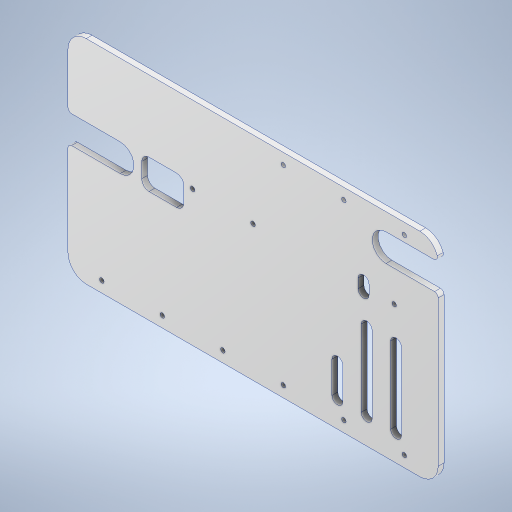
# Autodesk Inventor part: Class-D RevA Board Heatsink
Saved by Autodesk Inventor 2024 (Build 280153000, 153)
## iProperties
Created: 2023-08-05
Part Number: Class-D RevA Board Heatsink
Material: Aluminum 6061
Document SubType Name: Modeling
Designer: Ishaan
Density: 2.7 g/cm^3
Appearance: Aluminum - Flat
Author: Ishaan
Autodesk Inventor part; units mm, degrees
ref_plane "YZ Plane" through (0, 0, 0) normal (1, 0, 0) x (0, 1, 0)
ref_plane "XZ Plane" through (0, 0, 0) normal (0, 1, 0) x (-1, 0, 0)
ref_plane "XY Plane" through (0, 0, 0) normal (0, 0, 1) x (1, 0, 0)
sketch "Sketch1" plane through (0, 0, 0) normal (0, 0, 1) x (1, 0, 0)
  line L0 (-99, -56) -> (99, -56)
  line L1 (99, -56) -> (99, 56)
  line L2 (99, 56) -> (-99, 56)
  line L3 (-99, 56) -> (-99, -56)
  line L4 (-99, -56) -> (99, 56) construction
  line L5 (99, -56) -> (-99, 56) construction
  line L6 (-99, -56) -> (8.25, -56)
  line L7 (8.25, -56) -> (8.25, 20)
  line L8 (8.25, 20) -> (-99, 20)
  line L9 (-99, 20) -> (-99, -56)
  line L10 (8.25, 20) -> (8.25, 56)
  point P0 (0, 0)
  dimension "d0" = 112
  dimension "d1" = 198
  dimension "d3" = 76
  dimension "d50" = 8.25
  constraints: 22 end point, 4 parallel, 3 perpendicular, 2 horizontal, 2 midpoint, 1 point on line
  measures "d0" distance of L0.end L1.end
  measures "d1" distance of L1.end L2.end
  measures "d3" distance of L6.end L7.end
  measures "d50" distance from line of L10 point (0, 0)
extrude "Extrusion1" add sketch "Sketch1" along normal blind 3.175
sketch "Sketch2" plane through (0, 0, 3.175) normal (0, 0, 1) x (1, 0, 0)
  line L0 (-99, -56) -> (99, -56) projected
  line L1 (-99, 56) -> (-99, -56) projected
  line L2 (99, 56) -> (-99, 56) projected
  line L3 (99, -56) -> (99, 56) projected
  line L4 (-16.5, -52) -> (16.5, -52) construction
  line L5 (-49.5, -52) -> (-16.5, -52) construction
  line L6 (8.25, 20) -> (-99, 20) projected
  point P0 (0, 0)
  point P1 (-82.5, -52)
  point P2 (49.5, -52)
  point P3 (-82.5, 52)
  point P4 (-49.5, 52)
  point P5 (-16.5, 52)
  point P6 (16.5, 52)
  point P7 (49.5, 52)
  point P8 (82.5, -52)
  point P9 (82.5, 52)
  point P10 (-33, 16)
  point P11 (0, 16)
  point P12 (0, -52)
  point P13 (-33, -52)
  dimension "d6" = 4
  dimension "d9" = 33
  dimension "d12" = 104
  dimension "d15" = 4
  dimension "d17" = 16.5
  dimension "d18" = 16.5
  dimension "d51" = 4
  constraints: 4 end point, 3 horizontal, 2 midpoint, 2 vertical alignment, 1 coincident, 1 horizontal alignment, 1 vertical, 11 other
  measures "d6" distance from line of point (-82.5, -52) L0
  measures "d9" distance of point (-82.5, -52) L5.start
  measures "d12" distance of point (-82.5, -52) point (-82.5, 52)
  measures "d15" distance from line of L2 point (-82.5, 52)
  measures "d17" distance from line of point (-82.5, -52) L1
  measures "d18" distance from line of point (82.5, -52) L3
  measures "d51" distance from line of L6 point (-33, 16)
hole "Hole1" at (-82.5, -52, 3.175) at (-49.5, -52, 3.175) at (-16.5, -52, 3.175) at (16.5, -52, 3.175) at (49.5, -52, 3.175) at (16.5, 52, 3.175) at (49.5, 52, 3.175) at (82.5, -52, 3.175) at (82.5, 52, 3.175) at (-33, 16, 3.175) at (0, 16, 3.175) direction (0, 0, -1) diameter 2.459 end through all thread size "M3x0.5" class "6H" standard "ANSI Metric M Profile"
fillet "Fillet4" radius 8 4 edges at (99, -56, 1.5875) (-99, -56, 1.5875) (-99, 56, 1.5875) (99, 56, 1.5875)
sketch "Sketch6" plane through (0, 0, 3.175) normal (0, 0, 1) x (1, 0, 0)
  arc A0 (99, 48) -> (91, 56) centre (91, 48) ccw projected
  line L0 (91, 56) -> (-91, 56) projected
  arc A1 (-91, 56) -> (-99, 48) centre (-91, 48) ccw projected
  line L1 (-99, 48) -> (-99, -48) projected
  arc A2 (-99, -48) -> (-91, -56) centre (-91, -48) ccw projected
  line L2 (-91, -56) -> (91, -56) projected
  arc A3 (91, -56) -> (99, -48) centre (91, -48) ccw projected
  line L3 (99, -48) -> (99, 48) projected
  circle A4 centre (0, 16) radius 1.2295 projected
  circle A5 centre (-33, 16) radius 1.2295 projected
  circle A6 centre (82.5, 52) radius 1.2295 projected
  circle A7 centre (82.5, -52) radius 1.2295 projected
  circle A8 centre (49.5, 52) radius 1.2295 projected
  circle A9 centre (16.5, 52) radius 1.2295 projected
  circle A10 centre (49.5, -52) radius 1.2295 projected
  circle A11 centre (16.5, -52) radius 1.2295 projected
  circle A12 centre (-16.5, -52) radius 1.2295 projected
  circle A13 centre (-49.5, -52) radius 1.2295 projected
  circle A14 centre (-82.5, -52) radius 1.2295 projected
  line L4 (-91, 58) -> (91, 58)
  arc A15 (101, 48) -> (91, 58) centre (91, 48) ccw
  line L5 (101, 48) -> (101, -48)
  arc A16 (91, -58) -> (101, -48) centre (91, -48) ccw
  line L6 (91, -58) -> (-91, -58)
  arc A17 (-101, -48) -> (-91, -58) centre (-91, -48) ccw
  line L7 (-101, -48) -> (-101, 48)
  arc A18 (-91, 58) -> (-101, 48) centre (-91, 48) ccw
  point P0 (0, 0)
  dimension "d53" = 2
  constraints: 8 end point, 8 point on circle, 4 centre point, 7 other
  measures "d53" distance between parallel lines of L0 L4
extrude "Extrusion3" add sketch "Sketch6" against normal up to surface (3.175 mm away) contours L4 A15 L5 A16 L6 A17 L7 A18
sketch "Sketch7" plane through (0, 0, 0) normal (0, 0, -1) x (-1, 0, 0)
  circle A0 centre (-91.5, 41) radius 2.0701 projected
  circle A1 centre (-72.5, 41) radius 2.0701 projected
  circle A2 centre (72.5, 11) radius 2.0701 projected
  circle A3 centre (91.5, 11) radius 2.0701 projected
  line L0 (-72.5, 41) -> (-91.5, 41) construction
  line L1 (-72.5, 48.5) -> (-91.5, 48.5)
  line L2 (-91.5, 33.5) -> (-72.5, 33.5)
  arc A4 (-72.5, 33.5) -> (-72.5, 48.5) centre (-72.5, 41) ccw
  arc A5 (-91.5, 48.5) -> (-91.5, 33.5) centre (-91.5, 41) ccw
  line L3 (-91.5, 48.5) -> (-101, 48.5)
  line L4 (-101, 48.5) -> (-101, 33.5)
  line L5 (-101, 33.5) -> (-91.5, 33.5)
  line L6 (-91.5, 33.5) -> (-91.5, 48.5)
  line L7 (-101, 48) -> (-101, -48) projected
  line L8 (72.5, 11) -> (91.5, 11) construction
  line L9 (72.5, 3.5) -> (91.5, 3.5)
  line L10 (91.5, 18.5) -> (72.5, 18.5)
  arc A6 (72.5, 18.5) -> (72.5, 3.5) centre (72.5, 11) ccw
  arc A7 (91.5, 3.5) -> (91.5, 18.5) centre (91.5, 11) ccw
  line L11 (91.5, 18.5) -> (101, 18.5)
  line L12 (101, 18.5) -> (101, 3.5)
  line L13 (101, 3.5) -> (91.5, 3.5)
  line L14 (91.5, 3.5) -> (91.5, 18.5)
  line L15 (101, -48) -> (101, 48) projected
  point P0 (0, 0)
  point P1 (-82, 41)
  point P2 (82, 11)
  dimension "d56" = 15
  constraints: 32 end point, 8 point on circle, 8 tangent, 6 parallel, 4 centre point, 4 horizontal, 2 midpoint, 2 perpendicular, 1 collinear, 1 equal radius, 1 point on line
  measures "d56" diameter of A5
extrude "Extrusion4" cut sketch "Sketch7" against normal through all contours A0 L6 | A0 L6 L1 A4 L2 | L6 A0 | A0 L6 A5 | A5 L5 L4 L3 | A1 | A2 | A3 L14 | A3 L14 A7 | L14 A3 | A3 L14 L9 A6 L10 | L11 L12 L13 A7
sketch "Sketch8" plane through (0, 0, 0) normal (0, 0, -1) x (-1, 0, 0)
  circle A0 centre (56.75, 6.9) radius 0.75 projected
  circle A1 centre (41.75, 15.1) radius 0.75 projected
  circle A2 centre (-46, -43.54) radius 0.5 projected
  circle A3 centre (-46, -26.46) radius 0.5 projected
  circle A4 centre (-62, -43.54) radius 0.5 projected
  circle A5 centre (-62, -1.875) radius 0.5 projected
  circle A6 centre (-78, -43.54) radius 0.5 projected
  circle A7 centre (-78, -1.875) radius 0.5 projected
  line L0 (-78, -43.54) -> (-78, -1.875) construction
  line L1 (-75, -43.54) -> (-75, -1.875)
  line L2 (-81, -1.875) -> (-81, -43.54)
  arc A8 (-81, -43.54) -> (-75, -43.54) centre (-78, -43.54) ccw
  arc A9 (-75, -1.875) -> (-81, -1.875) centre (-78, -1.875) ccw
  line L3 (-62, -43.54) -> (-62, -1.875) construction
  line L4 (-59, -43.54) -> (-59, -1.875)
  line L5 (-65, -1.875) -> (-65, -43.54)
  arc A10 (-65, -43.54) -> (-59, -43.54) centre (-62, -43.54) ccw
  arc A11 (-59, -1.875) -> (-65, -1.875) centre (-62, -1.875) ccw
  line L6 (-46, -43.54) -> (-46, -26.46) construction
  line L7 (-49, -43.54) -> (-49, -26.46)
  line L8 (-43, -26.46) -> (-43, -43.54)
  arc A12 (-49, -43.54) -> (-43, -43.54) centre (-46, -43.54) ccw
  arc A13 (-43, -26.46) -> (-49, -26.46) centre (-46, -26.46) ccw
  line L9 (41.75, 19.1) -> (56.75, 19.1)
  line L10 (60.75, 15.1) -> (60.75, 6.9)
  line L11 (56.75, 2.9) -> (41.75, 2.9)
  line L12 (37.75, 6.9) -> (37.75, 15.1)
  arc A14 (41.75, 19.1) -> (37.75, 15.1) centre (41.75, 15.1) ccw
  arc A15 (56.75, 2.9) -> (60.75, 6.9) centre (56.75, 6.9) ccw
  arc A16 (60.75, 15.1) -> (56.75, 19.1) centre (56.75, 15.1) ccw
  arc A17 (37.75, 6.9) -> (41.75, 2.9) centre (41.75, 6.9) ccw
  circle A18 centre (-60.27, 19.04) radius 0.55 projected
  circle A19 centre (-60.27, 13.96) radius 0.55 projected
  line L13 (-60.27, 19.04) -> (-60.27, 13.96) construction
  line L14 (-63.27, 19.04) -> (-63.27, 13.96)
  line L15 (-57.27, 13.96) -> (-57.27, 19.04)
  arc A20 (-57.27, 19.04) -> (-63.27, 19.04) centre (-60.27, 19.04) ccw
  arc A21 (-63.27, 13.96) -> (-57.27, 13.96) centre (-60.27, 13.96) ccw
  point P0 (0, 0)
  point P1 (-78, -22.7075)
  point P2 (-62, -22.7075)
  point P3 (-46, -35)
  point P4 (-60.27, 16.5)
  dimension "d59" = 3
  dimension "d60" = 4
  constraints: 40 end point, 24 point on circle, 24 tangent, 12 centre point, 8 parallel, 6 equal radius, 4 midpoint, 2 concentric, 2 vertical, 1 horizontal, 1 perpendicular
  measures "d59" radius of A9
  measures "d60" radius of A14
extrude "Extrusion5" cut sketch "Sketch8" against normal through all contours A0 | A1 | A2 | A3 | A4 | A5 | A6 | A7 | A8 L2 A9 L1 | A10 L5 A11 L4 | L7 A13 L8 A12 | L9 A16 L10 A15 L11 A17 L12 A14 | A18 | A19 | A20 L15 A21 L14
sketch "Sketch9" plane through (0, 0, 3.175) normal (0, 0, 1) x (1, 0, 0)
  circle A0 centre (76.975, 16.5) radius 1.8675 projected
  point P0 (0, 0)
hole "Hole3" at (76.975, 16.5, 3.175) direction (0, 0, -1) diameter 2.459 end through all thread size "M3x0.5" class "6H" standard "ANSI Metric M Profile"
fillet "Fillet5" radius 2 4 edges at (-101, 18.5, 1.5875) (-101, 3.5, 1.5875) (100.9875, 48.5, 1.5875) (101, 33.5, 1.5875)
sketch "Sketch10" plane through (0, 0, 3.175) normal (0, 0, 1) x (1, 0, 0)
  circle A0 centre (76.975, 16.5) radius 1.2295 projected
  line L0 (65, -1.875) -> (65, -43.54) projected
  arc A1 (59, -43.54) -> (65, -43.54) centre (62, -43.54) ccw projected
  line L1 (59, -43.54) -> (59, -1.875) projected
  arc A2 (65, -1.875) -> (59, -1.875) centre (62, -1.875) ccw projected
  line L2 (81, -1.875) -> (81, -43.54) projected
  arc A3 (75, -43.54) -> (81, -43.54) centre (78, -43.54) ccw projected
  line L3 (75, -43.54) -> (75, -1.875) projected
  arc A4 (81, -1.875) -> (75, -1.875) centre (78, -1.875) ccw projected
  arc A5 (-60.75, 6.9) -> (-56.75, 2.9) centre (-56.75, 6.9) ccw projected
  line L4 (-60.75, 6.9) -> (-60.75, 15.1) projected
  arc A6 (-56.75, 19.1) -> (-60.75, 15.1) centre (-56.75, 15.1) ccw projected
  line L5 (-56.75, 19.1) -> (-41.75, 19.1) projected
  arc A7 (-37.75, 15.1) -> (-41.75, 19.1) centre (-41.75, 15.1) ccw projected
  line L6 (-37.75, 15.1) -> (-37.75, 6.9) projected
  arc A8 (-41.75, 2.9) -> (-37.75, 6.9) centre (-41.75, 6.9) ccw projected
  line L7 (-41.75, 2.9) -> (-56.75, 2.9) projected
  arc A9 (43, -43.54) -> (49, -43.54) centre (46, -43.54) ccw projected
  line L8 (43, -43.54) -> (43, -26.46) projected
  arc A10 (49, -26.46) -> (43, -26.46) centre (46, -26.46) ccw projected
  line L9 (49, -26.46) -> (49, -43.54) projected
  line L10 (57.27, 13.96) -> (57.27, 19.04) projected
  arc A11 (63.27, 19.04) -> (57.27, 19.04) centre (60.27, 19.04) ccw projected
  line L11 (63.27, 19.04) -> (63.27, 13.96) projected
  arc A12 (57.27, 13.96) -> (63.27, 13.96) centre (60.27, 13.96) ccw projected
  circle A13 centre (-82.5, -52) radius 1.2295 projected
  circle A14 centre (-49.5, -52) radius 1.2295 projected
  circle A15 centre (-16.5, -52) radius 1.2295 projected
  circle A16 centre (16.5, -52) radius 1.2295 projected
  circle A17 centre (49.5, -52) radius 1.2295 projected
  circle A18 centre (16.5, 52) radius 1.2295 projected
  circle A19 centre (49.5, 52) radius 1.2295 projected
  circle A20 centre (82.5, -52) radius 1.2295 projected
  circle A21 centre (82.5, 52) radius 1.2295 projected
  circle A22 centre (-33, 16) radius 1.2295 projected
  circle A23 centre (0, 16) radius 1.2295 projected
  arc A24 (101, 31.5) -> (99, 33.5) centre (99, 31.5) ccw projected
  line L12 (99, 33.5) -> (72.5, 33.5) projected
  arc A25 (72.5, 48.5) -> (72.5, 33.5) centre (72.5, 41) ccw projected
  line L13 (72.5, 48.5) -> (98.5993, 48.5) projected
  arc A26 (98.5993, 48.5) -> (100.4992, 51.125) centre (98.5993, 50.5) ccw projected
  arc A27 (100.4992, 51.125) -> (91, 58) centre (91, 48) ccw projected
  line L14 (91, 58) -> (-91, 58) projected
  arc A28 (-91, 58) -> (-101, 48) centre (-91, 48) ccw projected
  line L15 (-101, 48) -> (-101, 20.5) projected
  arc A29 (-101, 20.5) -> (-99, 18.5) centre (-99, 20.5) ccw projected
  line L16 (-99, 18.5) -> (-72.5, 18.5) projected
  arc A30 (-72.5, 3.5) -> (-72.5, 18.5) centre (-72.5, 11) ccw projected
  line L17 (-72.5, 3.5) -> (-99, 3.5) projected
  arc A31 (-99, 3.5) -> (-101, 1.5) centre (-99, 1.5) ccw projected
  line L18 (-101, 1.5) -> (-101, -48) projected
  arc A32 (-101, -48) -> (-91, -58) centre (-91, -48) ccw projected
  line L19 (-91, -58) -> (91, -58) projected
  arc A33 (91, -58) -> (101, -48) centre (91, -48) ccw projected
  line L20 (101, -48) -> (101, 31.5) projected
  point P0 (0, 0)
sketch "Sketch3" plane through (0, 0, 3.175) normal (0, 0, 1) x (1, 0, 0)
  circle A0 centre (0, 16) radius 1.7 projected
  circle A1 centre (-33, 16) radius 1.7 projected
  circle A2 centre (82.5, 52) radius 1.7 projected
  circle A3 centre (82.5, -52) radius 1.7 projected
  circle A4 centre (49.5, 52) radius 1.7 projected
  circle A5 centre (16.5, 52) radius 1.7 projected
  circle A6 centre (49.5, -52) radius 1.7 projected
  circle A7 centre (16.5, -52) radius 1.7 projected
  circle A8 centre (-16.5, -52) radius 1.7 projected
  circle A9 centre (-49.5, -52) radius 1.7 projected
  circle A10 centre (-82.5, -52) radius 1.7 projected
  line L0 (99, 56) -> (-99, 56) projected
  line L1 (-99, 56) -> (-99, -56) projected
  line L2 (-99, -56) -> (99, -56) projected
  line L3 (99, -56) -> (99, 56) projected
  line L4 (99, 23) -> (0, 23) construction
  line L5 (99, 10) -> (-99, 10) construction
  line L6 (90.5, -56) -> (90.5, 10)
  line L7 (99, 23) -> (80.5, 23)
  line L8 (80.5, 23) -> (80.5, 10)
  line L9 (90.5, 10) -> (80.5, 10)
  line L10 (63.5, 10) -> (80.5, 10)
  line L11 (80.5, 10) -> (80.5, 23)
  line L12 (80.5, 23) -> (63.5, 23)
  line L13 (63.5, 23) -> (63.5, 10)
  line L14 (63.5, 10) -> (80.5, 23) construction
  line L15 (80.5, 10) -> (63.5, 23) construction
  point P0 (0, 0)
  point P1 (82.5, 27)
  point P2 (72, 16.5)
  dimension "d29" = 4
  dimension "d30" = 8
  dimension "d31" = 4
  dimension "d32" = 4
  dimension "d33" = 2
  dimension "d36" = 72.5
  dimension "d37" = 17
  dimension "d38" = 13
  constraints: 24 end point, 8 point on line, 3 perpendicular, 2 collinear, 2 midpoint, 2 parallel, 2 vertical, 1 horizontal, 1 vertical alignment
  measures "d29" distance from line of L2 A3.centre
  measures "d30" distance from line of L6 A3.centre
  measures "d31" distance from line of L4 point (82.5, 27)
  measures "d32" distance from line of L0 A2.centre
  measures "d33" distance from line of L8 point (82.5, 27)
  measures "d36" distance from line of L2 point (72, 16.5)
  measures "d37" distance between parallel lines of L8 L13
  measures "d38" distance between parallel lines of L12 L10
equation "\"d15\" = d6"
equation "\"d18\" = d17"
equation "\"d31\" = d32"
body "Solid1"
